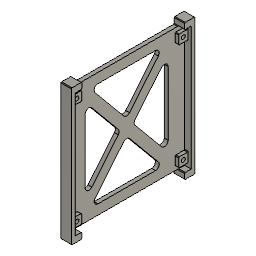
main_assembly (Autodesk Fusion 360 archive; units mm, degrees)
design "frame_Y±"
part number: 2026-06-25-10-46-33-182
Autodesk Fusion 360 part; units mm, degrees
note: some values were not read from the file. Chosen so that the rebuilt part matches the saved one: a direction. Set by a fixed rule: which sketch regions a step uses.
imported_body "Source Assembly: MASTER_ASSEMBLY_new" makes body 1
sketch "Sketch1" plane through (0, 0, 0) normal (0, 0, 1) x (1, 0, 0)
  line L0 (0, 0) -> (0, -100) construction
  line L1 (2, 0) -> (8.5, 0)
  line L2 (8.5, 0) -> (8.5, -3.2)
  line L3 (3.2, -8.5) -> (0, -8.5)
  line L4 (0, -8.5) -> (0, -2)
  line L5 (2, -100) -> (8.5, -100)
  line L6 (8.5, -100) -> (8.5, -96.8)
  line L7 (3.2, -91.5) -> (0, -91.5)
  line L8 (0, -91.5) -> (0, -98)
  line L9 (3.2, -8.5) -> (3.2, -3.2)
  line L10 (3.2, -3.2) -> (8.5, -3.2)
  line L11 (3.2, -91.5) -> (3.2, -96.8)
  line L12 (3.2, -96.8) -> (8.5, -96.8)
  line L13 (0, -8.5) -> (3.2, -8.5)
  line L14 (3.2, -8.5) -> (3.2, -91.5)
  line L15 (0, -91.5) -> (0, -8.5)
  line L16 (2, 0) -> (0, 0)
  line L17 (0, -2) -> (0, 0)
  line L18 (0, -98) -> (0, -100)
  line L19 (0, -100) -> (2, -100)
  dimension "d65" = 100
  dimension "d66" = 8.5
  dimension "d67" = 8.5
  dimension "d68" = 8.5
  dimension "d69" = 8.5
  dimension "d76" = 3.2
  dimension "d111" = 3.2
  dimension "d112" = 3.2
  constraint vertical L0
  constraint coincident L0.start L16.end
  constraint horizontal L1
  constraint vertical L2
  constraint horizontal L3
  constraint vertical L4
  constraint horizontal L5
  constraint vertical L6
  constraint horizontal L7
  constraint vertical L8
  constraint vertical L9
  constraint horizontal L10
  constraint vertical L11
  constraint horizontal L12
  constraint coincident L0.start L1
  constraint coincident L0.start L4
  constraint coincident L0.end L5
  constraint coincident L0.end L8
  constraint horizontal L13
  constraint vertical L14
  constraint vertical L15
  constraint equal L11 L12
  constraint equal L9 L10
  measures "d65" distance of L0.start L0.end
  measures "d66" distance of L0.start L1.end
  measures "d67" distance of L0.start L3.end
  measures "d68" distance of L0.end L5.end
  measures "d69" distance of L0.end L7.end
  measures "d76" distance of L3.end L3.start
  measures "d111" distance of L4 L9
  measures "d112" distance of L8 L11
extrude "Extrude1" add sketch "Sketch1" along normal blind 100 separate body makes body 2
sketch "Sketch5" plane through (0, 0, 0) normal (1, 0, 0) x (0, 1, 0)
  line L0 (-91.5, 0) -> (-8.5, 0)
  line L1 (-8.5, 0) -> (-8.5, 100)
  line L2 (-8.5, 100) -> (-91.5, 100)
  line L3 (-91.5, 100) -> (-91.5, 0)
  line L4 (-91.5, 100) -> (-8.5, 0) construction
  line L5 (-8.5, 100) -> (-91.5, 0) construction
  line L6 (-91.5, 50) -> (-8.5, 50) construction
  line L7 (-50, 100) -> (-50, 0) construction
  line L8 (-75.5814, 87.084) -> (-52.3084, 59.0443)
  line L9 (-73.273, 92) -> (-26.727, 92)
  line L10 (-24.4186, 87.084) -> (-47.6916, 59.0443)
  line L11 (-78.1916, 77.7027) -> (-56.7886, 51.916)
  line L12 (-83.5, 75.7867) -> (-83.5, 24.2133)
  line L13 (-78.1916, 22.2973) -> (-56.7886, 48.084)
  arc A0 (-73.273, 92) -> (-75.5814, 87.084) centre (-73.273, 89) ccw
  arc A1 (-78.1916, 77.7027) -> (-83.5, 75.7867) centre (-80.5, 75.7867) ccw
  arc A2 (-83.5, 24.2133) -> (-78.1916, 22.2973) centre (-80.5, 24.2133) ccw
  arc A3 (-56.7886, 48.084) -> (-56.7886, 51.916) centre (-59.097, 50) ccw
  arc A4 (-52.3084, 59.0443) -> (-47.6916, 59.0443) centre (-50, 60.9603) ccw
  arc A5 (-24.4186, 87.084) -> (-26.727, 92) centre (-26.727, 89) ccw
  line L14 (-24.4186, 12.916) -> (-47.6916, 40.9557)
  arc A6 (-26.727, 8) -> (-24.4186, 12.916) centre (-26.727, 11) ccw
  line L15 (-73.273, 8) -> (-26.727, 8)
  arc A7 (-75.5814, 12.916) -> (-73.273, 8) centre (-73.273, 11) ccw
  line L16 (-75.5814, 12.916) -> (-52.3084, 40.9557)
  arc A8 (-47.6916, 40.9557) -> (-52.3084, 40.9557) centre (-50, 39.0397) ccw
  line L17 (-21.8084, 77.7027) -> (-43.2114, 51.916)
  arc A9 (-43.2114, 51.916) -> (-43.2114, 48.084) centre (-40.903, 50) ccw
  line L18 (-21.8084, 22.2973) -> (-43.2114, 48.084)
  line L19 (-16.5, 75.7867) -> (-16.5, 24.2133)
  arc A10 (-21.8084, 22.2973) -> (-16.5, 24.2133) centre (-19.5, 24.2133) ccw
  arc A11 (-16.5, 75.7867) -> (-21.8084, 77.7027) centre (-19.5, 75.7867) ccw
  line L20 (0, 0) -> (-100, 0)
  line L21 (-100, 100) -> (0, 100)
  line L22 (-100, 0) -> (-100, 100)
  line L23 (0, 100) -> (0, 0)
  dimension "d78" = 8
  dimension "d79" = 8
  dimension "d80" = 4
  dimension "d81" = 4
  dimension "d82" = 3
  dimension "d83" = 3
  dimension "d84" = 3
  dimension "d85" = 3
  dimension "d86" = 3
  dimension "d87" = 3
  constraint coincident L2.end L3.start
  constraint coincident L0.end L1.start
  constraint coincident L1.end L2.start
  constraint coincident L0.start L3.end
  constraint midpoint L3 L6.start
  constraint midpoint L1 L6.end
  constraint midpoint L2 L7.start
  constraint midpoint L0 L7.end
  constraint perpendicular L7 L9
  constraint parallel L4 L11
  constraint parallel L4 L8
  constraint parallel L5 L10
  constraint parallel L5 L13
  constraint vertical L12
  constraint tangent L8 A0
  constraint tangent L9 A0
  constraint tangent L11 A1
  constraint tangent L12 A1
  constraint tangent L12 A2
  constraint tangent L13 A2
  constraint tangent L11 A3
  constraint tangent L13 A3
  constraint tangent L8 A4
  constraint tangent L10 A4
  constraint tangent L9 A5
  constraint tangent L10 A5
  constraint coincident L7 A4.centre
  constraint coincident L6 A3.centre
  constraint symmetric L6 L8.start A7.start
  constraint symmetric L6 L9.start L15.start
  constraint symmetric L6 A0 A7
  constraint symmetric L6 L8.end L16.end
  constraint symmetric L6 L10.end L14.end
  constraint symmetric L6 A4 A8
  constraint symmetric L6 L9.end A6.start
  constraint symmetric L6 L10.start L14.start
  constraint symmetric L6 A5 A6
  constraint symmetric L7 L11.start L17.start
  constraint symmetric L7 L12.start L19.start
  constraint symmetric L7 A1 A11
  constraint symmetric L7 L12.end L19.end
  constraint symmetric L7 L13.start L18.start
  constraint symmetric L7 A2 A10
  constraint symmetric L7 L11.end L17.end
  constraint symmetric L7 L13.end A9.end
  constraint symmetric L7 A3 A9
  measures "d78" distance of L3 L12
  measures "d79" distance of L2 L9
  measures "d80" distance of L4 L8
  measures "d81" distance of L4 L11
  measures "d82" radius of A0
  measures "d83" radius of A1
  measures "d84" radius of A2
  measures "d85" radius of A3
  measures "d86" radius of A4
  measures "d87" radius of A5
extrude "Extrude3" cut sketch "Sketch5" along normal blind 3.2 contours L8 L9 L10 A0 A4 A5 | L11 L12 L13 A1 A2 A3 | L14 A6 L15 A7 L16 A8 | L17 A9 L18 L19 A10 A11 bodies 2
sketch "Sketch7" plane through (0, 0, 100) normal (0, 0, 1) x (-1, 0, 0)
  line L0 (0, 100) -> (-8.5, 100)
  line L1 (-8.5, 100) -> (-8.5, 96.8)
  line L2 (-8.5, 96.8) -> (-3.2, 96.8)
  line L3 (-3.2, 96.8) -> (-3.2, 3.2)
  line L4 (-3.2, 3.2) -> (-8.5, 3.2)
  line L5 (-8.5, 3.2) -> (-8.5, 0)
  line L6 (-8.5, 0) -> (0, 0)
  line L7 (0, 0) -> (0, 100)
  line L8 (-8.5, 100) -> (-2, 100)
  line L9 (0, 98) -> (0, 91.5)
  line L10 (0, 91.5) -> (-8.5, 91.5)
  line L11 (-8.5, 91.5) -> (-8.5, 100)
  line L12 (-8.5, 0) -> (-2, 0)
  line L13 (0, 2) -> (0, 8.5)
  line L14 (0, 8.5) -> (-8.5, 8.5)
  line L15 (-8.5, 8.5) -> (-8.5, 0)
  line L16 (-2, 0) -> (0, 0)
  line L17 (0, 2) -> (0, 0)
  line L18 (0, 98) -> (0, 100)
  line L19 (-2, 100) -> (0, 100)
  point P0 (0, 100)
  dimension "d113" = 8.5
  dimension "d114" = 8.5
  dimension "d116" = 8.5
  dimension "d117" = 8.5
  constraint horizontal L8
  constraint vertical L9
  constraint horizontal L10
  constraint vertical L11
  constraint coincident L0.end L1.start
  constraint coincident P0 L8
  constraint coincident P0 L9
  constraint horizontal L12
  constraint vertical L13
  constraint horizontal L14
  constraint vertical L15
  constraint coincident L5.end L6.start
  constraint coincident L6.end L12
  constraint coincident L6.end L13
  constraint coincident L6.end L7.start
  constraint coincident P0 L0.start
  measures "d113" distance of L0.end P0
  measures "d114" distance of L0.end L10.end
  measures "d116" distance of L5.end L6.end
  measures "d117" distance of L5.end L14.end
extrude "Extrude6" add sketch "Sketch7" along normal blind 5 contours L0 L1 L2 L3 L7 L8 L9 L10 L11 L18 L19 | L2 L3 L10 L11 | L3 L4 L5 L6 L7 L12 L13 L14 L15 L16 L17 | L3 L4 L14 L15 bodies 2
sketch "Sketch8" plane through (0, 0, 0) normal (0, 0, -1) x (1, 0, 0)
  line L0 (0, 100) -> (0, 0)
  line L1 (0, 0) -> (8.5, 0)
  line L2 (8.5, 0) -> (8.5, 3.2)
  line L3 (8.5, 3.2) -> (3.2, 3.2)
  line L4 (3.2, 3.2) -> (3.2, 96.8)
  line L5 (3.2, 96.8) -> (8.5, 96.8)
  line L6 (8.5, 96.8) -> (8.5, 100)
  line L7 (8.5, 100) -> (0, 100)
  line L8 (8.5, 0) -> (2.1, 0)
  line L9 (0, 2.1) -> (0, 8.5)
  line L10 (0, 8.5) -> (8.5, 8.5)
  line L11 (8.5, 8.5) -> (8.5, 0)
  line L12 (8.5, 100) -> (2, 100)
  line L13 (0, 98) -> (0, 91.5)
  line L14 (0, 91.5) -> (8.5, 91.5)
  line L15 (8.5, 91.5) -> (8.5, 100)
  line L16 (2.1, 0) -> (0, 0)
  line L17 (0, 2.1) -> (0, 0)
  line L18 (2, 100) -> (0, 100)
  line L19 (0, 98) -> (0, 100)
  point P0 (0, 100)
  dimension "d121" = 8.5
  dimension "d122" = 8.5
  dimension "d123" = 8.5
  dimension "d124" = 8.5
  constraint horizontal L8
  constraint vertical L9
  constraint horizontal L10
  constraint vertical L11
  constraint coincident L1.end L2.start
  constraint horizontal L12
  constraint vertical L13
  constraint horizontal L14
  constraint vertical L15
  constraint coincident L6.end L7.start
  constraint coincident P0 L12
  constraint coincident P0 L13
  constraint coincident L0.end L8
  constraint coincident L0.end L9
  constraint coincident L0.end L1.start
  constraint coincident P0 L0.start
  measures "d121" distance of L1.end L0.end
  measures "d122" distance of L1.end L10.end
  measures "d123" distance of L6.end P0
  measures "d124" distance of L6.end L14.end
extrude "Extrude7" add sketch "Sketch8" along normal blind 5 contours L0 L4 L5 L6 L7 L12 L13 L14 L15 L18 L19 | L0 L1 L2 L3 L4 L8 L9 L10 L11 L16 L17 | L4 L5 L14 L15 | L3 L4 L10 L11 bodies 2
move_body "Move1" bodies 2 to x (1, 0, 0) y (0, 1, 0) z (0, 0, 1) at (0, 0, 10)
sketch "Sketch15" plane through (3.2, 0, 0) normal (1, 0, 0) x (0, 1, 0)
  line L0 (-73.273, 102) -> (-26.727, 102)
  arc A0 (-24.4186, 97.084) -> (-26.727, 102) centre (-26.727, 99) ccw
  line L1 (-24.4186, 97.084) -> (-47.6916, 69.0443)
  arc A1 (-52.3084, 69.0443) -> (-47.6916, 69.0443) centre (-50, 70.9603) ccw
  line L2 (-52.3084, 69.0443) -> (-75.5814, 97.084)
  arc A2 (-73.273, 102) -> (-75.5814, 97.084) centre (-73.273, 99) ccw
  line L3 (-21.8084, 32.2973) -> (-43.2114, 58.084)
  arc A3 (-43.2114, 61.916) -> (-43.2114, 58.084) centre (-40.903, 60) ccw
  line L4 (-43.2114, 61.916) -> (-21.8084, 87.7027)
  arc A4 (-16.5, 85.7867) -> (-21.8084, 87.7027) centre (-19.5, 85.7867) ccw
  line L5 (-16.5, 85.7867) -> (-16.5, 34.2133)
  arc A5 (-21.8084, 32.2973) -> (-16.5, 34.2133) centre (-19.5, 34.2133) ccw
  line L6 (-78.1916, 87.7027) -> (-56.7886, 61.916)
  arc A6 (-56.7886, 58.084) -> (-56.7886, 61.916) centre (-59.097, 60) ccw
  line L7 (-56.7886, 58.084) -> (-78.1916, 32.2973)
  arc A7 (-83.5, 34.2133) -> (-78.1916, 32.2973) centre (-80.5, 34.2133) ccw
  line L8 (-83.5, 34.2133) -> (-83.5, 85.7867)
  arc A8 (-78.1916, 87.7027) -> (-83.5, 85.7867) centre (-80.5, 85.7867) ccw
  line L9 (-75.5814, 22.916) -> (-52.3084, 50.9557)
  arc A9 (-47.6916, 50.9557) -> (-52.3084, 50.9557) centre (-50, 49.0397) ccw
  line L10 (-47.6916, 50.9557) -> (-24.4186, 22.916)
  arc A10 (-26.727, 18) -> (-24.4186, 22.916) centre (-26.727, 21) ccw
  line L11 (-26.727, 18) -> (-73.273, 18)
  arc A11 (-75.5814, 22.916) -> (-73.273, 18) centre (-73.273, 21) ccw
  line L12 (-8.5, 10) -> (-3.2, 10)
  line L13 (-3.2, 10) -> (-3.2, 110)
  line L14 (-3.2, 110) -> (-8.5, 110)
  line L15 (-8.5, 110) -> (-91.5, 110)
  line L16 (-91.5, 110) -> (-96.8, 110)
  line L17 (-96.8, 110) -> (-96.8, 10)
  line L18 (-96.8, 10) -> (-91.5, 10)
  line L19 (-91.5, 10) -> (-8.5, 10)
  line L20 (-96.8, 13.2) -> (-89.2, 13.2)
  line L21 (-89.2, 13.2) -> (-89.2, 20.8)
  line L22 (-89.2, 20.8) -> (-96.8, 20.8)
  line L23 (-96.8, 20.8) -> (-96.8, 13.2)
  line L24 (-89.2, 17) -> (-93, 17) construction
  line L25 (-3.2, 13.2) -> (-10.8, 13.2)
  line L26 (-10.8, 13.2) -> (-10.8, 20.8)
  line L27 (-10.8, 20.8) -> (-3.2, 20.8)
  line L28 (-3.2, 20.8) -> (-3.2, 13.2)
  line L29 (-10.8, 17) -> (-7, 17) construction
  line L30 (-3.2, 106.8) -> (-10.8, 106.8)
  line L31 (-10.8, 106.8) -> (-10.8, 99.2)
  line L32 (-10.8, 99.2) -> (-3.2, 99.2)
  line L33 (-3.2, 99.2) -> (-3.2, 106.8)
  line L34 (-96.8, 106.8) -> (-89.2, 106.8)
  line L35 (-89.2, 106.8) -> (-89.2, 99.2)
  line L36 (-89.2, 99.2) -> (-96.8, 99.2)
  line L37 (-96.8, 99.2) -> (-96.8, 106.8)
  line L38 (-96.8, 103) -> (-93, 103) construction
  line L39 (-3.2, 103) -> (-7, 103) construction
  dimension "d213" = 3.2
  dimension "d214" = 7.6
  dimension "d215" = 7.6
  dimension "d216" = 3.8
  dimension "d218" = 7.6
  dimension "d219" = 7.6
  dimension "d220" = 3.2
  dimension "d221" = 3.8
  dimension "d222" = 7.6
  dimension "d224" = 3.2
  dimension "d225" = 7.6
  dimension "d226" = 7.6
  dimension "d227" = 7.6
  dimension "d228" = 3.2
  constraint horizontal L20
  constraint vertical L21
  constraint horizontal L22
  constraint vertical L23
  constraint coincident L17 L20.start
  constraint midpoint L21 L24.start
  constraint perpendicular L21 L24
  constraint horizontal L25
  constraint vertical L26
  constraint horizontal L27
  constraint vertical L28
  constraint coincident L13 L25.start
  constraint midpoint L26 L29.start
  constraint perpendicular L26 L29
  constraint horizontal L30
  constraint vertical L31
  constraint horizontal L32
  constraint vertical L33
  constraint coincident L13 L30.start
  constraint horizontal L34
  constraint vertical L35
  constraint horizontal L36
  constraint vertical L37
  constraint coincident L17 L34.start
  constraint midpoint L37 L38.start
  constraint perpendicular L17 L38
  constraint midpoint L33 L39.start
  constraint perpendicular L13 L39
  measures "d213" distance of L18 L20
  measures "d214" distance of L21 L23
  measures "d215" distance of L20.end L21.end
  measures "d216" distance of L24.start L24.end
  measures "d218" distance of L26.end L27.end
  measures "d219" distance of L25.end L26.end
  measures "d220" distance of L12 L25
  measures "d221" distance of L29.start L29.end
  measures "d222" distance of L30.start L32.end
  measures "d224" distance of L14 L30
  measures "d225" distance of L31.end L32.end
  measures "d226" distance of L34.start L34.end
  measures "d227" distance of L34.start L36.end
  measures "d228" distance of L16 L34
sketch "Sketch16" plane through (0, 0, 0) normal (-1, 0, 0) x (0, -1, 0)
  line L0 (26.727, 102) -> (73.273, 102)
  arc A0 (75.5814, 97.084) -> (73.273, 102) centre (73.273, 99) ccw
  line L1 (75.5814, 97.084) -> (52.3084, 69.0443)
  arc A1 (47.6916, 69.0443) -> (52.3084, 69.0443) centre (50, 70.9603) ccw
  line L2 (47.6916, 69.0443) -> (24.4186, 97.084)
  arc A2 (26.727, 102) -> (24.4186, 97.084) centre (26.727, 99) ccw
  line L3 (43.2114, 58.084) -> (21.8084, 32.2973)
  arc A3 (16.5, 34.2133) -> (21.8084, 32.2973) centre (19.5, 34.2133) ccw
  line L4 (16.5, 34.2133) -> (16.5, 85.7867)
  arc A4 (21.8084, 87.7027) -> (16.5, 85.7867) centre (19.5, 85.7867) ccw
  line L5 (21.8084, 87.7027) -> (43.2114, 61.916)
  arc A5 (43.2114, 58.084) -> (43.2114, 61.916) centre (40.903, 60) ccw
  line L6 (56.7886, 61.916) -> (78.1916, 87.7027)
  arc A6 (83.5, 85.7867) -> (78.1916, 87.7027) centre (80.5, 85.7867) ccw
  line L7 (83.5, 85.7867) -> (83.5, 34.2133)
  arc A7 (78.1916, 32.2973) -> (83.5, 34.2133) centre (80.5, 34.2133) ccw
  line L8 (78.1916, 32.2973) -> (56.7886, 58.084)
  arc A8 (56.7886, 61.916) -> (56.7886, 58.084) centre (59.097, 60) ccw
  line L9 (52.3084, 50.9557) -> (75.5814, 22.916)
  arc A9 (73.273, 18) -> (75.5814, 22.916) centre (73.273, 21) ccw
  line L10 (73.273, 18) -> (26.727, 18)
  arc A10 (24.4186, 22.916) -> (26.727, 18) centre (26.727, 21) ccw
  line L11 (24.4186, 22.916) -> (47.6916, 50.9557)
  arc A11 (52.3084, 50.9557) -> (47.6916, 50.9557) centre (50, 49.0397) ccw
  line L12 (0, 5) -> (8.5, 5)
  line L13 (8.5, 5) -> (8.5, 10)
  line L14 (8.5, 10) -> (91.5, 10)
  line L15 (91.5, 10) -> (91.5, 5)
  line L16 (100, 115) -> (91.5, 115)
  line L17 (91.5, 115) -> (91.5, 110)
  line L18 (91.5, 110) -> (8.5, 110)
  line L19 (8.5, 110) -> (8.5, 115)
  line L20 (100, 5) -> (100, 115)
  line L21 (0, 115) -> (0, 5)
  line L22 (91.5, 5) -> (100, 5)
  line L23 (8.5, 115) -> (0, 115)
  point P0 (93, 17)
  point P1 (93, 103)
  point P2 (7, 103)
  point P3 (7, 17)
extrude "Extrude11" add sketch "Sketch15" along normal blind 2.8 contours L13 L25 L26 L27 L28 | L17 L20 L21 L22 L23 | L13 L30 L31 L32 L33 | L17 L34 L35 L36 L37 bodies 2
hole "Hole1" at (0, -93, 103) at (0, -7, 103) at (0, -7, 17) at (0, -93, 17) direction (1, 0, 0) diameter 3.2 depth 10 tip angle 180 counterbore diameter 6 counterbore depth 3 bodies 2
fillet "Fillet4" radius 0.5 16 edges at (1.6, -91.5, 110) (4.25, -91.5, 115) (4.25, -100, 115) (4.25, 0, 115) (4.25, -8.5, 115) (1.6, -8.5, 110) (1.6, -8.5, 10) (4.25, -8.5, 5) (4.25, 0, 5) (4.25, -100, 5) (1.6, -91.5, 10) (4.25, -91.5, 5) (5.85, -91.5, 10) (5.85, -8.5, 10) (5.85, -91.5, 110) (5.85, -8.5, 110) on bodies 2
fillet "Fillet5" radius 0.5 12 edges at (4.6, -89.2, 106.8) (4.6, -89.2, 99.2) (4.6, -10.8, 106.8) (4.6, -10.8, 99.2) (4.6, -3.2, 99.2) (4.6, -96.8, 99.2) (4.6, -96.8, 20.8) (4.6, -89.2, 20.8) (4.6, -89.2, 13.2) (4.6, -10.8, 13.2) (4.6, -10.8, 20.8) (4.6, -3.2, 20.8) on bodies 2
hidden bodies 1
equation "d11 = MAX_h_w"
equation "rail_width = 8.5 mm"
equation "rail_wall_thickness = wall_thickness"
equation "wall_thickness = 3.2 mm"
equation "rib_width = 8 mm"
equation "rib_fillet = 3 mm"
equation "d66 = rail_width"
equation "d67 = rail_width"
equation "d68 = rail_width"
equation "d69 = rail_width"
equation "d76 = wall_thickness"
equation "MAX_h_w = 100 mm"
equation "d78 = rib_width"
equation "d79 = rib_width"
equation "d80 = rib_width / 2"
equation "d81 = rib_width / 2"
equation "d82 = rib_fillet"
equation "d83 = rib_fillet"
equation "d84 = rib_fillet"
equation "d85 = rib_fillet"
equation "d86 = rib_fillet"
equation "d87 = rib_fillet"
equation "d88 = wall_thickness"
equation "m3_insert_depth = 5 mm"
equation "m3_insert_diameter = 4.4 mm"
equation "d111 = rail_wall_thickness"
equation "d112 = rail_wall_thickness"
equation "d113 = rail_width"
equation "d114 = rail_width"
equation "d116 = rail_width"
equation "d117 = rail_width"
equation "d121 = rail_width"
equation "d122 = rail_width"
equation "d123 = rail_width"
equation "d124 = rail_width"
equation "rail_fillet = 2 mm"
equation "m3_insert_radius = m3_insert_diameter / 2"
equation "insert_tolerance = 1.6 mm"
equation "d213 = wall_thickness"
equation "d214 = m3_insert_diameter + 2 * insert_tolerance"
equation "d215 = m3_insert_diameter + 2 * insert_tolerance"
equation "d216 = m3_insert_radius + insert_tolerance"
equation "d218 = m3_insert_diameter + 2 * insert_tolerance"
equation "d219 = m3_insert_diameter + 2 * insert_tolerance"
equation "d220 = wall_thickness"
equation "d221 = m3_insert_radius + insert_tolerance"
equation "d222 = m3_insert_diameter + 2 * insert_tolerance"
equation "d224 = wall_thickness"
equation "d225 = m3_insert_diameter + 2 * insert_tolerance"
equation "d226 = m3_insert_diameter + 2 * insert_tolerance"
equation "d227 = m3_insert_diameter + 2 * insert_tolerance"
equation "d228 = wall_thickness"
equation "d229 = 11 mm - wall_thickness - m3_insert_depth"
named bodies: "Body3 (MASTER_ASSEMBLY_new)"

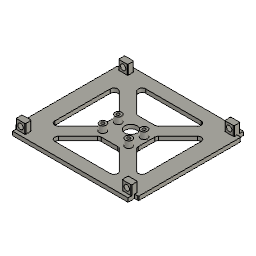
design "frame_Z-"
part number: 2026-06-25-14-04-03-692
Autodesk Fusion 360 part; units mm, degrees
sketch "Sketch3" plane through (0, 0, 0) normal (0, 0, 1) x (1, 0, 0)
  line L0 (0, 0) -> (100, 0)
  line L1 (100, 0) -> (100, 93.6)
  line L2 (100, 93.6) -> (0, 93.6)
  line L3 (0, 93.6) -> (0, 0)
  line L4 (0, 93.6) -> (3.2, 93.6)
  line L5 (3.2, 93.6) -> (3.2, 88.3)
  line L6 (3.2, 88.3) -> (0, 88.3)
  line L7 (0, 88.3) -> (0, 93.6)
  line L8 (100, 93.6) -> (96.8, 93.6)
  line L9 (96.8, 93.6) -> (96.8, 88.3)
  line L10 (96.8, 88.3) -> (100, 88.3)
  line L11 (100, 88.3) -> (100, 93.6)
  line L12 (100, 0) -> (96.8, 0)
  line L13 (96.8, 0) -> (96.8, 5.3)
  line L14 (96.8, 5.3) -> (100, 5.3)
  line L15 (100, 5.3) -> (100, 0)
  line L16 (0, 0) -> (3.2, 0)
  line L17 (3.2, 0) -> (3.2, 5.3)
  line L18 (3.2, 5.3) -> (0, 5.3)
  line L19 (0, 5.3) -> (0, 0)
  line L20 (3.2, 93.6) -> (96.8, 0) construction
  line L21 (96.8, 93.6) -> (3.2, 0) construction
  line L22 (0, 46.8) -> (50, 46.8) construction
  line L23 (25.3924, 78.4787) -> (41.1924, 62.6787)
  line L24 (58.8076, 62.6787) -> (74.6076, 78.4787)
  line L25 (72.4863, 83.6) -> (27.5137, 83.6)
  arc A0 (27.5137, 83.6) -> (25.3924, 78.4787) centre (27.5137, 80.6) ccw
  arc A1 (74.6076, 78.4787) -> (72.4863, 83.6) centre (72.4863, 80.6) ccw
  line L26 (43.3137, 61.8) -> (56.6863, 61.8)
  arc A2 (41.1924, 62.6787) -> (43.3137, 61.8) centre (43.3137, 64.8) ccw
  arc A3 (56.6863, 61.8) -> (58.8076, 62.6787) centre (56.6863, 64.8) ccw
  line L27 (35, 40.1137) -> (35, 53.4863)
  arc A4 (34.1213, 37.9924) -> (35, 40.1137) centre (32, 40.1137) ccw
  line L28 (18.3213, 22.1924) -> (34.1213, 37.9924)
  arc A5 (13.2, 24.3137) -> (18.3213, 22.1924) centre (16.2, 24.3137) ccw
  line L29 (13.2, 69.2863) -> (13.2, 24.3137)
  line L30 (34.1213, 55.6076) -> (18.3213, 71.4076)
  arc A6 (35, 53.4863) -> (34.1213, 55.6076) centre (32, 53.4863) ccw
  arc A7 (18.3213, 71.4076) -> (13.2, 69.2863) centre (16.2, 69.2863) ccw
  line L31 (56.6863, 31.8) -> (43.3137, 31.8)
  arc A8 (58.8076, 30.9213) -> (56.6863, 31.8) centre (56.6863, 28.8) ccw
  line L32 (74.6076, 15.1213) -> (58.8076, 30.9213)
  arc A9 (72.4863, 10) -> (74.6076, 15.1213) centre (72.4863, 13) ccw
  line L33 (27.5137, 10) -> (72.4863, 10)
  line L34 (41.1924, 30.9213) -> (25.3924, 15.1213)
  arc A10 (43.3137, 31.8) -> (41.1924, 30.9213) centre (43.3137, 28.8) ccw
  arc A11 (25.3924, 15.1213) -> (27.5137, 10) centre (27.5137, 13) ccw
  line L35 (65, 53.4863) -> (65, 40.1137)
  arc A12 (65.8787, 55.6076) -> (65, 53.4863) centre (68, 53.4863) ccw
  line L36 (81.6787, 71.4076) -> (65.8787, 55.6076)
  arc A13 (86.8, 69.2863) -> (81.6787, 71.4076) centre (83.8, 69.2863) ccw
  line L37 (86.8, 24.3137) -> (86.8, 69.2863)
  line L38 (65.8787, 37.9924) -> (81.6787, 22.1924)
  arc A14 (65, 40.1137) -> (65.8787, 37.9924) centre (68, 40.1137) ccw
  arc A15 (81.6787, 22.1924) -> (86.8, 24.3137) centre (83.8, 24.3137) ccw
  circle A16 centre (50, 49.3) radius 5
  line L39 (50, 46.8) -> (50, 49.3) construction
  dimension "d53" = 100
  dimension "d54" = 93.6
  dimension "d55" = 3.2
  dimension "d56" = 5.3
  dimension "d57" = 3.2
  dimension "d58" = 5.3
  dimension "d59" = 5.3
  dimension "d60" = 3.2
  dimension "d61" = 3.2
  dimension "d62" = 5.3
  dimension "d64" = 5
  dimension "d65" = 5
  dimension "d66" = 10
  dimension "d67" = 3
  dimension "d68" = 3
  dimension "d116" = 3
  dimension "d118" = 360
  dimension "d135" = 10
  dimension "d137" = 15
  dimension "d144" = 2.5
  constraint horizontal L0
  constraint vertical L1
  constraint horizontal L2
  constraint vertical L3
  constraint coincident L0.start L3.end
  constraint horizontal L4
  constraint vertical L5
  constraint horizontal L6
  constraint vertical L7
  constraint horizontal L8
  constraint vertical L9
  constraint horizontal L10
  constraint vertical L11
  constraint horizontal L12
  constraint vertical L13
  constraint horizontal L14
  constraint vertical L15
  constraint horizontal L16
  constraint vertical L17
  constraint horizontal L18
  constraint vertical L19
  constraint midpoint L3 L22.start
  constraint midpoint L20 L22.end
  constraint horizontal L25
  constraint parallel L20 L23
  constraint parallel L21 L24
  constraint tangent L23 A0
  constraint tangent L25 A0
  constraint tangent L24 A1
  constraint tangent L25 A1
  constraint tangent L23 A2
  constraint tangent L26 A2
  constraint tangent L24 A3
  constraint tangent L26 A3
  constraint equal A2 A3
  constraint horizontal L26
  constraint perpendicular L22 L39
  constraint coincident A16.centre L39.end
  measures "d53" distance of L0.start L0.end
  measures "d54" distance of L0.start L2.end
  measures "d55" distance of L2.end L4.end
  measures "d56" distance of L2.end L6.end
  measures "d57" distance of L1.end L8.end
  measures "d58" distance of L1.end L10.end
  measures "d59" distance of L0.end L14.end
  measures "d60" distance of L1 L13
  measures "d61" distance of L0.start L16.end
  measures "d62" distance of L0.start L18.end
  measures "d64" distance of L20 L23
  measures "d65" distance of L21 L24
  measures "d66" distance of L2 L25
  measures "d67" radius of A0
  measures "d68" radius of A1
  measures "d116" radius of A2
  measures "d135" diameter of A16
  measures "d137" distance of L22.end L26
  measures "d144" distance of L22.end A16.centre
extrude "Extrude3" add sketch "Sketch3" along normal blind 3.2 contours L0 L1 L2 L3 L5 L6 L9 L10 L13 L14 L17 L18
sketch "Sketch4" plane through (0, 0, 3.2) normal (0, 0, 1) x (-1, 0, 0)
  line L0 (-41.1924, -62.6787) -> (-25.3924, -78.4787)
  arc A0 (-27.5137, -83.6) -> (-25.3924, -78.4787) centre (-27.5137, -80.6) ccw
  line L1 (-27.5137, -83.6) -> (-72.4863, -83.6)
  arc A1 (-74.6076, -78.4787) -> (-72.4863, -83.6) centre (-72.4863, -80.6) ccw
  line L2 (-74.6076, -78.4787) -> (-58.8076, -62.6787)
  line L3 (-3.2, 0) -> (-96.8, 0)
  line L4 (-96.8, 0) -> (-96.8, -5.3)
  line L5 (-96.8, -5.3) -> (-100, -5.3)
  line L6 (-100, -5.3) -> (-100, -88.3)
  line L7 (-100, -88.3) -> (-96.8, -88.3)
  line L8 (-96.8, -88.3) -> (-96.8, -93.6)
  line L9 (-96.8, -93.6) -> (-3.2, -93.6)
  line L10 (-3.2, -93.6) -> (-3.2, -88.3)
  line L11 (-3.2, -88.3) -> (0, -88.3)
  line L12 (0, -88.3) -> (0, -5.3)
  line L13 (0, -5.3) -> (-3.2, -5.3)
  line L14 (-3.2, -5.3) -> (-3.2, 0)
  line L15 (-3.2, -90.8) -> (-10.8, -90.8)
  line L16 (-10.8, -90.8) -> (-10.8, -85.8)
  line L17 (-10.8, -85.8) -> (-3.2, -85.8)
  line L18 (-3.2, -85.8) -> (-3.2, -90.8)
  line L19 (-96.8, -90.8) -> (-89.2, -90.8)
  line L20 (-89.2, -90.8) -> (-89.2, -85.8)
  line L21 (-89.2, -85.8) -> (-96.8, -85.8)
  line L22 (-96.8, -85.8) -> (-96.8, -90.8)
  line L23 (-96.8, -2.8) -> (-89.2, -2.8)
  line L24 (-89.2, -2.8) -> (-89.2, -7.8)
  line L25 (-89.2, -7.8) -> (-96.8, -7.8)
  line L26 (-96.8, -7.8) -> (-96.8, -2.8)
  line L27 (-3.2, -2.8) -> (-10.8, -2.8)
  line L28 (-10.8, -2.8) -> (-10.8, -7.8)
  line L29 (-10.8, -7.8) -> (-3.2, -7.8)
  line L30 (-3.2, -7.8) -> (-3.2, -2.8)
  arc A2 (-25.3924, -15.1213) -> (-27.5137, -10) centre (-27.5137, -13) ccw
  line L31 (-25.3924, -15.1213) -> (-41.1924, -30.9213)
  arc A3 (-43.3137, -31.8) -> (-41.1924, -30.9213) centre (-43.3137, -28.8) ccw
  line L32 (-43.3137, -31.8) -> (-56.6863, -31.8)
  arc A4 (-58.8076, -30.9213) -> (-56.6863, -31.8) centre (-56.6863, -28.8) ccw
  line L33 (-58.8076, -30.9213) -> (-74.6076, -15.1213)
  arc A5 (-72.4863, -10) -> (-74.6076, -15.1213) centre (-72.4863, -13) ccw
  line L34 (-72.4863, -10) -> (-27.5137, -10)
  arc A6 (-18.3213, -71.4076) -> (-13.2, -69.2863) centre (-16.2, -69.2863) ccw
  line L35 (-18.3213, -71.4076) -> (-34.1213, -55.6076)
  arc A7 (-35, -53.4863) -> (-34.1213, -55.6076) centre (-32, -53.4863) ccw
  line L36 (-35, -53.4863) -> (-35, -40.1137)
  arc A8 (-34.1213, -37.9924) -> (-35, -40.1137) centre (-32, -40.1137) ccw
  line L37 (-34.1213, -37.9924) -> (-18.3213, -22.1924)
  arc A9 (-13.2, -24.3137) -> (-18.3213, -22.1924) centre (-16.2, -24.3137) ccw
  line L38 (-13.2, -24.3137) -> (-13.2, -69.2863)
  arc A10 (-81.6787, -22.1924) -> (-86.8, -24.3137) centre (-83.8, -24.3137) ccw
  line L39 (-81.6787, -22.1924) -> (-65.8787, -37.9924)
  arc A11 (-65, -40.1137) -> (-65.8787, -37.9924) centre (-68, -40.1137) ccw
  line L40 (-65, -40.1137) -> (-65, -53.4863)
  arc A12 (-65.8787, -55.6076) -> (-65, -53.4863) centre (-68, -53.4863) ccw
  line L41 (-65.8787, -55.6076) -> (-81.6787, -71.4076)
  arc A13 (-86.8, -69.2863) -> (-81.6787, -71.4076) centre (-83.8, -69.2863) ccw
  line L42 (-86.8, -69.2863) -> (-86.8, -24.3137)
  arc A14 (-56.6863, -61.8) -> (-58.8076, -62.6787) centre (-56.6863, -64.8) ccw
  line L43 (-56.6863, -61.8) -> (-43.3137, -61.8)
  arc A15 (-41.1924, -62.6787) -> (-43.3137, -61.8) centre (-43.3137, -64.8) ccw
  circle A16 centre (-50, -49.3) radius 5
  dimension "d74" = 2.8
  dimension "d76" = 7.6
  dimension "d77" = 5
  dimension "d80" = 7.6
  dimension "d81" = 5
  dimension "d82" = 2.8
  dimension "d83" = 7.6
  dimension "d84" = 5
  dimension "d85" = 2.8
  dimension "d86" = 7.6
  dimension "d87" = 5
  dimension "d88" = 2.8
  constraint horizontal L15
  constraint vertical L16
  constraint horizontal L17
  constraint vertical L18
  constraint coincident L10 L15.start
  constraint horizontal L19
  constraint vertical L20
  constraint horizontal L21
  constraint vertical L22
  constraint coincident L8 L19.start
  constraint horizontal L23
  constraint vertical L24
  constraint horizontal L25
  constraint vertical L26
  constraint coincident L4 L23.start
  constraint horizontal L27
  constraint vertical L28
  constraint horizontal L29
  constraint vertical L30
  constraint coincident L14 L27.start
  measures "d74" distance of L9 L15
  measures "d76" distance of L16 L18
  measures "d77" distance of L15 L17
  measures "d80" distance of L19.start L19.end
  measures "d81" distance of L19.start L21.end
  measures "d82" distance of L9 L19
  measures "d83" distance of L23.start L23.end
  measures "d84" distance of L23.start L25.end
  measures "d85" distance of L3 L23
  measures "d86" distance of L27.start L27.end
  measures "d87" distance of L27.start L29.end
  measures "d88" distance of L3 L27
extrude "Extrude4" add sketch "Sketch4" along normal blind 7.6 contours L14 L27 L28 L29 L30 | L4 L23 L24 L25 L26 | L10 L15 L16 L17 L18 | L8 L19 L20 L21 L22
fillet "Fillet4" radius 0.5 20 edges at (3.2, 85.8, 7) (10.8, 85.8, 7) (3.2, 90.8, 7) (10.8, 90.8, 7) (89.2, 90.8, 7) (96.8, 90.8, 7) (89.2, 85.8, 7) (3.2, 7.8, 7) (10.8, 7.8, 7) (3.2, 2.8, 7) (0, 5.3, 1.6) (0, 88.3, 1.6) (89.2, 7.8, 7) (96.8, 7.8, 7) (89.2, 2.8, 7) (10.8, 2.8, 7) (96.8, 2.8, 7) (100, 5.3, 1.6) (96.8, 85.8, 7) (100, 88.3, 1.6)
sketch "Sketch5" plane through (0, 85.8, 0) normal (0, -1, 0) x (1, 0, 0)
  line L0 (96.3, 10.8) -> (89.7, 10.8)
  circle A0 centre (93, 7) radius 2.2
  line L1 (96.3, 3.2) -> (96.3, 10.8)
  line L2 (89.7, 10.8) -> (89.7, 3.2)
  line L3 (89.7, 3.2) -> (96.3, 3.2)
  dimension "d119" = 4.4
  dimension "d121" = 3.8
  measures "d119" diameter of A0
  measures "d121" distance of L0 A0.centre
sketch "Sketch6" plane through (0, 85.8, 0) normal (0, -1, 0) x (1, 0, 0)
  line L0 (10.3, 10.8) -> (3.7, 10.8)
  circle A0 centre (7, 7) radius 2.2
  line L1 (10.3, 3.2) -> (10.3, 10.8)
  line L2 (3.7, 10.8) -> (3.7, 3.2)
  line L3 (3.7, 3.2) -> (10.3, 3.2)
  dimension "d122" = 4.4
  dimension "d123" = 3.8
  measures "d122" diameter of A0
  measures "d123" distance of L0 A0.centre
sketch "Sketch7" plane through (0, 7.8, 0) normal (0, 1, 0) x (-1, 0, 0)
  line L0 (-3.7, 10.8) -> (-10.3, 10.8)
  circle A0 centre (-7, 7) radius 2.2
  line L1 (-10.3, 10.8) -> (-10.3, 3.2)
  line L2 (-10.3, 3.2) -> (-3.7, 3.2)
  line L3 (-3.7, 3.2) -> (-3.7, 10.8)
  dimension "d125" = 4.4
  dimension "d127" = 3.8
  measures "d125" diameter of A0
  measures "d127" distance of L0 A0.centre
sketch "Sketch8" plane through (0, 7.8, 0) normal (0, 1, 0) x (-1, 0, 0)
  line L0 (-89.7, 10.8) -> (-96.3, 10.8)
  circle A0 centre (-93, 7) radius 2.2
  line L1 (-96.3, 10.8) -> (-96.3, 3.2)
  line L2 (-96.3, 3.2) -> (-89.7, 3.2)
  line L3 (-89.7, 3.2) -> (-89.7, 10.8)
  dimension "d128" = 4.4
  dimension "d129" = 3.8
  measures "d128" diameter of A0
  measures "d129" distance of L0 A0.centre
extrude "Extrude5" cut sketch "Sketch6" sketch "Sketch5" against normal blind 5 contours A0 of sketch 2 contours A0
extrude "Extrude6" cut sketch "Sketch8" sketch "Sketch7" against normal blind 5 contours A0 of sketch 2 contours A0
sketch "Sketch10" plane through (0, 0, 3.2) normal (0, 0, 1) x (-1, 0, 0)
  line L0 (-89.7, -90.8) -> (-96.3, -90.8)
  line L1 (-96.8, -88.3) -> (-96.8, -86.3)
  line L2 (-96.8, -93.6) -> (-3.2, -93.6)
  line L3 (-3.2, -5.3) -> (-3.2, -7.3)
  line L4 (-3.7, -90.8) -> (-10.3, -90.8)
  line L5 (-10.3, -2.8) -> (-3.7, -2.8)
  line L6 (-3.2, 0) -> (-96.8, 0)
  line L7 (-96.3, -2.8) -> (-89.7, -2.8)
  arc A0 (-25.3924, -15.1213) -> (-27.5137, -10) centre (-27.5137, -13) ccw
  line L8 (-25.3924, -15.1213) -> (-41.1924, -30.9213)
  arc A1 (-43.3137, -31.8) -> (-41.1924, -30.9213) centre (-43.3137, -28.8) ccw
  line L9 (-43.3137, -31.8) -> (-56.6863, -31.8)
  arc A2 (-58.8076, -30.9213) -> (-56.6863, -31.8) centre (-56.6863, -28.8) ccw
  line L10 (-58.8076, -30.9213) -> (-74.6076, -15.1213)
  arc A3 (-72.4863, -10) -> (-74.6076, -15.1213) centre (-72.4863, -13) ccw
  line L11 (-72.4863, -10) -> (-27.5137, -10)
  arc A4 (-18.3213, -71.4076) -> (-13.2, -69.2863) centre (-16.2, -69.2863) ccw
  line L12 (-18.3213, -71.4076) -> (-34.1213, -55.6076)
  arc A5 (-35, -53.4863) -> (-34.1213, -55.6076) centre (-32, -53.4863) ccw
  line L13 (-35, -53.4863) -> (-35, -40.1137)
  arc A6 (-34.1213, -37.9924) -> (-35, -40.1137) centre (-32, -40.1137) ccw
  line L14 (-34.1213, -37.9924) -> (-18.3213, -22.1924)
  arc A7 (-13.2, -24.3137) -> (-18.3213, -22.1924) centre (-16.2, -24.3137) ccw
  line L15 (-13.2, -24.3137) -> (-13.2, -69.2863)
  arc A8 (-81.6787, -22.1924) -> (-86.8, -24.3137) centre (-83.8, -24.3137) ccw
  line L16 (-81.6787, -22.1924) -> (-65.8787, -37.9924)
  arc A9 (-65, -40.1137) -> (-65.8787, -37.9924) centre (-68, -40.1137) ccw
  line L17 (-65, -40.1137) -> (-65, -53.4863)
  arc A10 (-65.8787, -55.6076) -> (-65, -53.4863) centre (-68, -53.4863) ccw
  line L18 (-65.8787, -55.6076) -> (-81.6787, -71.4076)
  arc A11 (-86.8, -69.2863) -> (-81.6787, -71.4076) centre (-83.8, -69.2863) ccw
  line L19 (-86.8, -69.2863) -> (-86.8, -24.3137)
  arc A12 (-56.6863, -61.8) -> (-58.8076, -62.6787) centre (-56.6863, -64.8) ccw
  line L20 (-56.6863, -61.8) -> (-43.3137, -61.8)
  arc A13 (-41.1924, -62.6787) -> (-43.3137, -61.8) centre (-43.3137, -64.8) ccw
  line L21 (-41.1924, -62.6787) -> (-25.3924, -78.4787)
  arc A14 (-27.5137, -83.6) -> (-25.3924, -78.4787) centre (-27.5137, -80.6) ccw
  line L22 (-27.5137, -83.6) -> (-72.4863, -83.6)
  arc A15 (-74.6076, -78.4787) -> (-72.4863, -83.6) centre (-72.4863, -80.6) ccw
  line L23 (-74.6076, -78.4787) -> (-58.8076, -62.6787)
  circle A16 centre (-39.5, -36.9) radius 2.8
  circle A17 centre (-39.5, -36.9) radius 1.2
  line L24 (-50, -49.3) -> (-50, -32.4573) construction
  circle A18 centre (-60.5, -36.9) radius 2.8
  circle A19 centre (-60.5, -36.9) radius 1.2
  line L25 (-34.2541, -43.15) -> (-66.2541, -43.15) construction
  circle A20 centre (-39.5, -49.4) radius 2.8
  circle A21 centre (-39.5, -49.4) radius 1.2
  circle A22 centre (-60.5, -49.4) radius 1.2
  circle A23 centre (-60.5, -49.4) radius 2.8
  arc A24 (-3.7, -7.8) -> (-3.2, -7.3) centre (-3.7, -7.3) ccw
  line L26 (-3.7, -7.8) -> (-10.3, -7.8)
  arc A25 (-10.8, -7.3) -> (-10.3, -7.8) centre (-10.3, -7.3) ccw
  line L27 (-10.8, -7.3) -> (-10.8, -3.3)
  arc A26 (-10.3, -2.8) -> (-10.8, -3.3) centre (-10.3, -3.3) ccw
  arc A27 (-3.2, -3.3) -> (-3.7, -2.8) centre (-3.7, -3.3) ccw
  line L28 (-3.2, -93.6) -> (-3.2, -90.3)
  arc A28 (-96.3, -2.8) -> (-96.8, -3.3) centre (-96.3, -3.3) ccw
  arc A29 (-89.2, -3.3) -> (-89.7, -2.8) centre (-89.7, -3.3) ccw
  line L29 (-89.2, -3.3) -> (-89.2, -7.3)
  arc A30 (-89.7, -7.8) -> (-89.2, -7.3) centre (-89.7, -7.3) ccw
  line L30 (-89.7, -7.8) -> (-96.3, -7.8)
  arc A31 (-96.8, -7.3) -> (-96.3, -7.8) centre (-96.3, -7.3) ccw
  line L31 (-96.8, -7.3) -> (-96.8, -5.3)
  line L32 (-96.8, -5.3) -> (-99.5, -5.3)
  arc A32 (-99.5, -5.3) -> (-100, -5.8) centre (-99.5, -5.8) ccw
  line L33 (-100, -5.8) -> (-100, -87.8)
  arc A33 (-100, -87.8) -> (-99.5, -88.3) centre (-99.5, -87.8) ccw
  line L34 (-99.5, -88.3) -> (-96.8, -88.3)
  arc A34 (-96.3, -85.8) -> (-96.8, -86.3) centre (-96.3, -86.3) ccw
  line L35 (-96.3, -85.8) -> (-89.7, -85.8)
  arc A35 (-89.2, -86.3) -> (-89.7, -85.8) centre (-89.7, -86.3) ccw
  line L36 (-89.2, -86.3) -> (-89.2, -90.3)
  arc A36 (-89.7, -90.8) -> (-89.2, -90.3) centre (-89.7, -90.3) ccw
  arc A37 (-96.8, -90.3) -> (-96.3, -90.8) centre (-96.3, -90.3) ccw
  line L37 (-96.8, -90.3) -> (-96.8, -93.6)
  arc A38 (-3.7, -90.8) -> (-3.2, -90.3) centre (-3.7, -90.3) ccw
  arc A39 (-10.8, -90.3) -> (-10.3, -90.8) centre (-10.3, -90.3) ccw
  line L38 (-10.8, -90.3) -> (-10.8, -86.3)
  arc A40 (-10.3, -85.8) -> (-10.8, -86.3) centre (-10.3, -86.3) ccw
  line L39 (-10.3, -85.8) -> (-3.7, -85.8)
  arc A41 (-3.2, -86.3) -> (-3.7, -85.8) centre (-3.7, -86.3) ccw
  line L40 (-3.2, -88.3) -> (-0.5, -88.3)
  arc A42 (-0.5, -88.3) -> (0, -87.8) centre (-0.5, -87.8) ccw
  line L41 (0, -87.8) -> (0, -5.8)
  arc A43 (0, -5.8) -> (-0.5, -5.3) centre (-0.5, -5.8) ccw
  line L42 (-0.5, -5.3) -> (-3.2, -5.3)
  line L43 (-3.2, -86.3) -> (-3.2, -88.3)
  line L44 (-3.2, -3.3) -> (-3.2, 0)
  line L45 (-96.8, 0) -> (-96.8, -3.3)
  point P0 (-50, -49.3)
  dimension "d140" = 5.6
  dimension "d141" = 2.4
  dimension "d142" = 12.4
  dimension "d143" = 10.5
  dimension "d145" = 32
  dimension "d146" = 6.25
  constraint concentric A16 A17
  constraint coincident P0 L24.start
  constraint vertical L24
  constraint symmetric A16 L24 A18
  constraint symmetric A17 L24 A19
  constraint perpendicular L17 L25
  constraint symmetric A16 L25 A20
  constraint symmetric A17 L25 A21
  constraint symmetric A18 L25 A23
  constraint symmetric A19 L25 A22
  measures "d140" diameter of A16
  measures "d141" diameter of A17
  measures "d142" vertical distance of A16.centre P0
  measures "d143" distance of A16.centre L24
  measures "d145" distance of L25.start L25.end
  measures "d146" distance of A16.centre L25
extrude "Extrude7" add sketch "Sketch10" along normal blind 5.3 contours A16 | A18 | A20 | A23
extrude "Extrude8" cut 4 faces at (60.2506, 48.8515, 3.2) (60.2506, 36.3515, 3.2) (39.2506, 36.3515, 3.2) (39.2506, 48.8515, 3.2) along direction (0, 0, -1) blind 5
equation "m3_insert_depth = 5 mm"
equation "m3_insert_diameter = 4.4 mm"
equation "rail_width = 8.5 mm"
equation "wall_thickness = 3.2 mm"
equation "rib_width = 10 mm"
equation "rib_fillet = 3 mm"
equation "MAX_h_w = 100 mm"
equation "rail_fillet = 2 mm"
equation "d53 = MAX_h_w"
equation "d54 = MAX_h_w - 2 * wall_thickness"
equation "d55 = wall_thickness"
equation "d56 = rail_width - wall_thickness"
equation "d57 = wall_thickness"
equation "d58 = rail_width - wall_thickness"
equation "d59 = rail_width - wall_thickness"
equation "d60 = wall_thickness"
equation "d61 = wall_thickness"
equation "d62 = rail_width - wall_thickness"
equation "d64 = rib_width / 2"
equation "d65 = rib_width / 2"
equation "d66 = rib_width"
equation "d67 = rib_fillet"
equation "d68 = rib_fillet"
equation "d72 = wall_thickness"
equation "d74 = 11 mm - wall_thickness - m3_insert_depth"
equation "insert_clearance = 1.6 mm"
equation "d76 = m3_insert_diameter + 2 * insert_clearance"
equation "d77 = m3_insert_depth"
equation "d78 = m3_insert_diameter + 2 * insert_clearance"
equation "d80 = m3_insert_diameter + 2 * insert_clearance"
equation "d81 = m3_insert_depth"
equation "d82 = 11 mm - wall_thickness - m3_insert_depth"
equation "d83 = m3_insert_diameter + 2 * insert_clearance"
equation "d84 = m3_insert_depth"
equation "d85 = 11 mm - wall_thickness - m3_insert_depth"
equation "d86 = m3_insert_diameter + 2 * insert_clearance"
equation "d87 = m3_insert_depth"
equation "d88 = 11 mm - wall_thickness - m3_insert_depth"
equation "m3_insert_radius = m3_insert_diameter / 2"
equation "d116 = rib_fillet"
equation "d119 = m3_insert_diameter"
equation "d121 = m3_insert_radius + insert_clearance"
equation "d122 = m3_insert_diameter"
equation "d123 = m3_insert_radius + insert_clearance"
equation "d125 = m3_insert_diameter"
equation "d127 = m3_insert_radius + insert_clearance"
equation "d128 = m3_insert_diameter"
equation "d129 = m3_insert_radius + insert_clearance"
equation "d131 = -m3_insert_depth"
equation "d133 = -m3_insert_depth"
equation "d137 = 5 mm + rib_width"
equation "d147 = 8.5 mm - wall_thickness"
